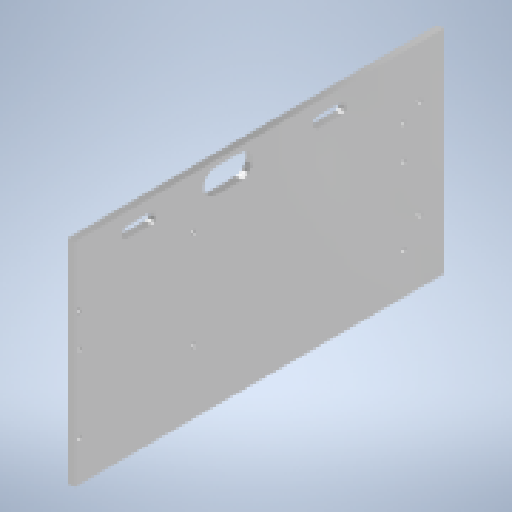
# Autodesk Inventor part: крышка
Saved by Autodesk Inventor 2024.2 (Build 282272000, 272)
## iProperties
Created: 2026-02-12
Part Number: крышка
Material: Типовые
Document SubType Name: Modeling
Designer: Service
Density: 1 g/cm^3
Appearance: Алюминий — плоский
Author: Service
Autodesk Inventor part; units mm, degrees
ref_plane "YZ Plane" through (0, 0, 0) normal (1, 0, 0) x (0, 1, 0)
ref_plane "XZ Plane" through (0, 0, 0) normal (0, 1, 0) x (-1, 0, 0)
ref_plane "XY Plane" through (0, 0, 0) normal (0, 0, 1) x (1, 0, 0)
sketch "Эскиз1" plane through (0, 0, 0) normal (1, 0, 0) x (0, 1, 0)
  line L0 (70.9825, 98.2222) -> (-59.0175, 98.2222)
  line L1 (-59.0175, 98.2222) -> (-59.0175, -105.7778)
  line L2 (-59.0175, -105.7778) -> (70.9825, -105.7778)
  line L3 (70.9825, -105.7778) -> (70.9825, 98.2222)
  circle A0 centre (-34.0175, 95.2222) radius 1.5
  circle A1 centre (-34.0175, -102.7778) radius 1.5
  circle A2 centre (12.9825, 95.2222) radius 1.5
  circle A3 centre (12.9825, -102.7778) radius 1.5
  circle A4 centre (32.9825, 95.2222) radius 1.5
  circle A5 centre (32.9825, -102.7778) radius 1.5
  line L4 (-59.0175, -105.7778) -> (70.9825, -105.7778)
  line L5 (70.9825, -105.7778) -> (70.9825, -127.7504)
  line L6 (70.9825, -127.7504) -> (-59.0175, -127.7504)
  line L7 (-59.0175, -127.7504) -> (-59.0175, -105.7778)
  point P0 (0, 0)
  dimension "d0" = 204
  dimension "d1" = 130
  dimension "d2" = 3
  dimension "d3" = 25
  dimension "d4" = 25
  dimension "d5" = 3
  dimension "d6" = 3
  dimension "d7" = 3
  dimension "d8" = 72
  dimension "d9" = 3
  dimension "d10" = 3
  dimension "d11" = 3
  dimension "d12" = 72
  dimension "d13" = 3
  dimension "d14" = 3
  dimension "d15" = 20
  dimension "d16" = 3
  dimension "d17" = 3
  dimension "d18" = 20
  constraints: 16 end point, 6 centre point, 4 parallel, 2 horizontal, 2 perpendicular, 1 equal radius
  measures "d0" distance of L2.end L0.start
  measures "d1" distance of L0.start L0.end
  measures "d2" diameter of A0
  measures "d3" distance from line of L1 A0.centre
  measures "d4" distance from line of L1 A1.centre
  measures "d5" distance from line of L0 A0.centre
  measures "d6" distance from line of L2 A1.centre
  measures "d7" diameter of A2
  measures "d8" distance from line of A2.centre L1
  measures "d9" distance from line of L0 A2.centre
  measures "d10" diameter of A3
  measures "d11" distance from line of A3.centre L2
  measures "d12" distance from line of L1 A3.centre
  measures "d13" diameter of A4
  measures "d14" distance from line of L0 A4.centre
  measures "d15" distance of A2.centre A4.centre
  measures "d16" diameter of A5
  measures "d17" distance from line of L2 A5.centre
  measures "d18" distance of A3.centre A5.centre
extrude "Выдавливание1" add sketch "Эскиз1" along normal blind 4
sketch "Эскиз2" plane through (0, 0, 0) normal (-1, 0, 0) x (0, 0, 1)
  circle A0 centre (-112.7504, -20.3037) radius 1.5
  circle A1 centre (25.0776, -20.3037) radius 1.5
  line L0 (98.2222, -59.0175) -> (-105.7778, -59.0175) projected
  circle A2 centre (-112.7504, 39.6963) radius 1.5
  circle A3 centre (25.0776, 39.6963) radius 1.5
  line L1 (98.2222, 70.9825) -> (98.2222, -59.0175) projected
  circle A4 centre (-102.7778, 12.9825) radius 1.5 projected
  line L2 (-105.7778, -59.0175) -> (-105.7778, 70.9825) projected
  line L3 (-105.7778, 70.9825) -> (98.2222, 70.9825) projected
  line L4 (-127.7504, -59.0175) -> (-127.7504, 70.9825) projected
  point P0 (0, 0)
  point P1 (98.2222, 5.9825)
  dimension "d21" = 137.828
  dimension "d22" = 3
  dimension "d23" = 3
  dimension "d26" = 3
  dimension "d27" = 3
  dimension "d28" = 137.828
  dimension "d29" = 60
  dimension "d30" = 60
  dimension "d37" = 31.2861
  dimension "d38" = 31.2861
  dimension "d47" = 15
  dimension "d48" = 15
  constraints: 4 centre point, 1 midpoint
  measures "d21" distance of A0.centre A1.centre
  measures "d22" diameter of A0
  measures "d23" diameter of A1
  measures "d26" diameter of A2
  measures "d27" diameter of A3
  measures "d28" distance of A3.centre A2.centre
  measures "d29" distance of A0.centre A2.centre
  measures "d30" distance of A1.centre A3.centre
  measures "d37" distance from line of L3 A3.centre
  measures "d38" distance from line of L3 A2.centre
  measures "d47" distance from line of L4 A0.centre
  measures "d48" distance from line of L4 A2.centre
extrude "Выдавливание2" cut sketch "Эскиз2" against normal blind 5 contours A0 | A1 | A2 | A3
sketch "Эскиз3" plane through (0, 0, 0) normal (-1, 0, 0) x (0, 0, 1)
  line L0 (11.8903, 60.0049) -> (-3.1097, 60.0049) construction
  line L1 (11.8903, 67.5049) -> (-3.1097, 67.5049)
  line L2 (-3.1097, 52.5049) -> (11.8903, 52.5049)
  arc A0 (11.8903, 52.5049) -> (11.8903, 67.5049) centre (11.8903, 60.0049) ccw
  arc A1 (-3.1097, 67.5049) -> (-3.1097, 52.5049) centre (-3.1097, 60.0049) ccw
  line L3 (65.5667, 60.0049) -> (51.5667, 60.0049) construction
  line L4 (65.5667, 63.2549) -> (51.5667, 63.2549)
  line L5 (51.5667, 56.7549) -> (65.5667, 56.7549)
  arc A2 (65.5667, 56.7549) -> (65.5667, 63.2549) centre (65.5667, 60.0049) ccw
  arc A3 (51.5667, 63.2549) -> (51.5667, 56.7549) centre (51.5667, 60.0049) ccw
  line L6 (-50.6502, 60.0049) -> (-64.6502, 60.0049) construction
  line L7 (-50.6502, 63.2549) -> (-64.6502, 63.2549)
  line L8 (-64.6502, 56.7549) -> (-50.6502, 56.7549)
  arc A4 (-50.6502, 56.7549) -> (-50.6502, 63.2549) centre (-50.6502, 60.0049) ccw
  arc A5 (-64.6502, 63.2549) -> (-64.6502, 56.7549) centre (-64.6502, 60.0049) ccw
  line L9 (35.934, -50.5903) -> (-109.1416, -50.5903) construction
  line L10 (35.934, -47.1293) -> (-109.1416, -47.1293)
  line L11 (-109.1416, -54.0514) -> (35.934, -54.0514)
  arc A6 (35.934, -54.0514) -> (35.934, -47.1293) centre (35.934, -50.5903) ccw
  arc A7 (-109.1416, -47.1293) -> (-109.1416, -54.0514) centre (-109.1416, -50.5903) ccw
  point P0 (0, 0)
  point P1 (4.3903, 60.0049)
  point P2 (58.5667, 60.0049)
  point P3 (-57.6502, 60.0049)
  point P4 (-36.6038, -50.5903)
  dimension "d39" = 14
  dimension "d40" = 14
  dimension "d41" = 6.5
  dimension "d42" = 6.5
  dimension "d43" = 15
  dimension "d44" = 15
  constraints: 32 end point, 16 point on circle, 16 tangent, 8 centre point, 4 horizontal, 4 midpoint, 4 parallel, 2 collinear
  measures "d39" distance of L4.start L4.end
  measures "d40" distance of L7.start L7.end
  measures "d41" distance between parallel lines of L5 L4
  measures "d42" distance between parallel lines of L8 L7
  measures "d43" distance between parallel lines of L2 L1
  measures "d44" distance of L1.start L1.end
extrude "Выдавливание3" cut sketch "Эскиз3" against normal through all
